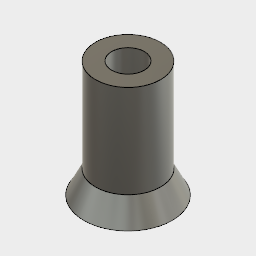
L5-PE-01 (Autodesk Fusion 360 design; units mm, degrees)
Autodesk Fusion 360 part; units mm, degrees
sketch "Sketch1" plane through (0, 0, 0) normal (0, 0, 1) x (1, 0, 0)
  line L0 (0, 0) -> (0, 50) construction
  line L1 (7, 50) -> (14, 50)
  line L2 (14, 50) -> (14, 10)
  line L3 (14, 10) -> (19, 0)
  line L4 (19, 0) -> (7, 0)
  line L5 (7, 0) -> (7, 50)
  line L6 (0, 47) -> (7, 47)
  line L7 (7, 47) -> (7, 50)
  line L8 (7, 50) -> (14, 50)
  line L9 (14, 50) -> (14, 44)
  line L10 (14, 44) -> (20, 44)
  line L11 (20, 44) -> (20, 47)
  arc A0 (20, 47) -> (10, 57) centre (10, 47) ccw
  line L12 (10, 57) -> (0, 57)
  line L13 (0, 57) -> (0, 47)
  dimension "d1" = 50
  dimension "d2" = 7
  dimension "d3" = 14
  dimension "d4" = 12
  dimension "d5" = 10
  dimension "d7" = 3
  dimension "d8" = 6
  dimension "d9" = 3
  dimension "d10" = 10
  dimension "d11" = 10
  dimension "d12" = 20
  measures "d1" distance of L0.start L0.end
  measures "d2" distance of L0 L5
  measures "d3" distance of L0 L2
  measures "d4" distance of L3.end L4.end
  measures "d5" distance of L0.start L2.end
  measures "d7" distance of L1.start L6.end
  measures "d8" distance of L1.end L10
  measures "d9" distance of L10.end L11.end
  measures "d10" radius of A0
  measures "d11" distance of L6.start L12.end
  measures "d12" distance of L11 L13
revolve "Revolve1" add sketch "Sketch1" angle 360 about axis through (0, 0, 0) along (0, 1, 0) contours L1 L2 L3 L4 L5 L7 L8 L9
